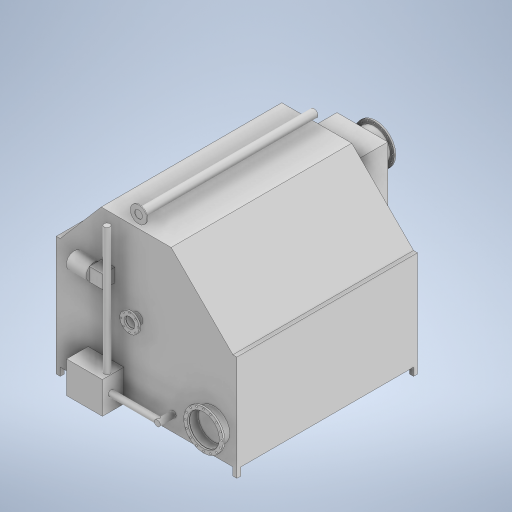
# Autodesk Inventor part: dummy
Saved by Autodesk Inventor 2023.1 (Build 271208000, 208)
## iProperties
Created: 2023-11-07
Part Number: dummy
Material: Generic
Document SubType Name: Modeling
Designer: admin
Density: 1 g/cm^3
Appearance: Default
Author: admin
Autodesk Inventor part; units mm, degrees
ref_plane "YZ Plane" through (0, 0, 0) normal (1, 0, 0) x (0, 1, 0)
ref_plane "XZ Plane" through (0, 0, 0) normal (0, 1, 0) x (-1, 0, 0)
ref_plane "XY Plane" through (0, 0, 0) normal (0, 0, 1) x (1, 0, 0)
sketch "Sketch1" plane through (0, 0, 0) normal (0, 0, 1) x (1, 0, 0)
  line L0 (-1135, 100) -> (1135, 100)
  line L1 (1135, 100) -> (1135, 1320)
  line L2 (1135, 1320) -> (-1135, 1320)
  line L3 (-1135, 1320) -> (-1135, 100)
  line L4 (-1135, 1320) -> (-1135, 1500)
  line L5 (-571.0934, 2100) -> (308.9066, 2100)
  line L6 (-1135, 1500) -> (-1085, 1500)
  line L7 (-1085, 1500) -> (-571.0934, 2100)
  line L8 (308.9066, 2100) -> (1085, 1320)
  point P0 (0, 0)
  point P1 (0, 100)
  dimension "d0" = 2270
  dimension "d1" = 100
  dimension "d2" = 1220
  dimension "d3" = 1400
  dimension "d4" = 880
  dimension "d5" = 50
  dimension "d6" = 50
  dimension "d7" = 2000
  dimension "d8" = 790
  dimension "d9" = 1100.3277
  constraints: 18 end point, 3 horizontal, 2 parallel, 1 midpoint, 1 perpendicular, 1 point on line, 1 vertical, 1 vertical alignment
  measures "d0" distance of L1.end L2.end
  measures "d1" distance from line of point (0, 0) L0
  measures "d2" distance of L0.end L1.end
  measures "d3" distance from line of L0 L4.end
  measures "d4" distance of L5.start L5.end
  measures "d5" distance of L4.end L6.end
  measures "d6" distance of L1.end L8.end
  measures "d7" distance between parallel lines of L0 L5
  measures "d8" distance of L6.end L5.start
  measures "d9" distance of L5.end L8.end
extrude "Extrusion1" add sketch "Sketch1" along normal mid plane 2270
sketch "Sketch2" plane through (-1135, 100, 1135) normal (0, -1, 0) x (1, 0, 0)
  line L0 (2270, -2270) -> (2270, 0) projected
  line L1 (0, 0) -> (2270, 0) projected
  line L2 (0, -2270) -> (0, 0) projected
  line L3 (2270, -2270) -> (0, -2270) projected
  line L4 (2270, 0) -> (2220, 0) projected
  line L5 (2270, 0) -> (2220, 0)
  line L6 (2220, 0) -> (2220, -50)
  line L7 (2220, -50) -> (2270, -50)
  line L8 (2270, -50) -> (2270, 0)
  line L9 (2220, -2270) -> (2270, -2270) projected
  line L10 (2270, -2270) -> (2220, -2270)
  line L11 (2220, -2270) -> (2220, -2220)
  line L12 (2220, -2220) -> (2270, -2220)
  line L13 (2270, -2220) -> (2270, -2270)
  line L14 (0, -2270) -> (50, -2270)
  line L15 (50, -2270) -> (50, -2220)
  line L16 (50, -2220) -> (0, -2220)
  line L17 (0, -2220) -> (0, -2270)
  line L18 (0, 0) -> (50, 0)
  line L19 (50, 0) -> (50, -50)
  line L20 (50, -50) -> (0, -50)
  line L21 (0, -50) -> (0, 0)
  line L22 (1160, -1110) -> (1110, -1110)
  line L23 (1110, -1110) -> (1110, -1160)
  line L24 (1110, -1160) -> (1160, -1160)
  line L25 (1160, -1160) -> (1160, -1110)
  line L26 (1160, -1110) -> (1110, -1160) construction
  line L27 (1110, -1110) -> (1160, -1160) construction
  point P0 (1135, -1135)
  point P1 (0, -2220)
  point P2 (50, -2270)
  dimension "d12" = 50
  dimension "d13" = 50
  constraints: 44 end point, 10 parallel, 8 equal length, 5 horizontal, 5 perpendicular, 2 midpoint, 1 point on line
  measures "d12" distance of L7.end L6.end
  measures "d13" distance of L5.end L6.end
extrude "Extrusion2" add sketch "Sketch2" along normal blind 100 contours L3 L11 L12 L0 | L7 L6 L1 L0 | L3 L2 L16 L15 | L19 L20 L2 L1 | L25 L24 L23 L22
sketch "Sketch3" plane through (0, 0, 1135) normal (0, 0, 1) x (1, 0, 0)
  circle A0 centre (845, 445) radius 200
  line L0 (-1085, 100) -> (1085, 100) projected
  circle A1 centre (845, 445) radius 195
  line L1 (1135, 1320) -> (1135, 0) projected
  line L2 (650, 640) -> (1040, 640) construction
  line L3 (1040, 640) -> (1040, 250) construction
  line L4 (1040, 250) -> (650, 250) construction
  line L5 (650, 250) -> (650, 640) construction
  point P0 (0, 0)
  point P1 (1135, 660)
  dimension "d18" = 400
  dimension "d19" = 390
  dimension "d20" = 95
  dimension "d21" = 485
  dimension "d22" = 150
  dimension "d23" = 540
  constraints: 8 end point, 4 tangent, 2 centre point, 2 parallel, 1 horizontal, 1 midpoint, 1 perpendicular
  measures "d18" diameter of A0
  measures "d19" diameter of A1
  measures "d20" distance between parallel lines of L1 L3
  measures "d21" distance from line of L5 point (1135, 660)
  measures "d22" distance between parallel lines of L0 L4
  measures "d23" distance between parallel lines of L0 L2
extrude "Extrusion3" add sketch "Sketch3" along normal blind 110
sketch "Sketch4" plane through (0, 0, 1135) normal (0, 0, 1) x (1, 0, 0)
  line L0 (1135, 1320) -> (1085, 1320) projected
  line L1 (1085, 1320) -> (308.9066, 2100) projected
  line L2 (308.9066, 2100) -> (-571.0934, 2100) projected
  line L3 (-571.0934, 2100) -> (-1085, 1500) projected
  line L4 (-1085, 1500) -> (-1135, 1500) projected
  line L5 (-1135, 1500) -> (-1135, 0) projected
  line L6 (-1085, 0) -> (-1135, 0) projected
  line L7 (-1085, 100) -> (-1085, 0) projected
  line L8 (-1085, 100) -> (1085, 100) projected
  line L9 (1085, 100) -> (1085, 0) projected
  line L10 (1135, 0) -> (1085, 0) projected
  line L11 (1135, 1320) -> (1135, 0) projected
  circle A0 centre (845, 445) radius 200 projected
  circle A1 centre (-115, 1120) radius 62.5
  line L12 (-177.5, 1182.5) -> (-52.5, 1182.5) construction
  line L13 (-52.5, 1182.5) -> (-52.5, 1057.5) construction
  line L14 (-52.5, 1057.5) -> (-177.5, 1057.5) construction
  line L15 (-177.5, 1057.5) -> (-177.5, 1182.5) construction
  circle A2 centre (-115, 1120) radius 67.5
  line L16 (25, 0) -> (-25, 0) projected
  point P0 (0, 0)
  point P1 (0, 0)
  dimension "d26" = 125
  dimension "d28" = 957.5
  dimension "d30" = 1312.5
  dimension "d31" = 5
  dimension "d134" = 1020
  dimension "d135" = 1120
  constraints: 8 end point, 4 tangent, 2 centre point, 2 parallel, 1 horizontal, 1 midpoint, 1 perpendicular
  measures "d26" diameter of A1
  measures "d28" distance between parallel lines of L8 L14
  measures "d30" distance between parallel lines of L11 L15
  measures "d31" radial gap between concentric circles of A1 A2
  measures "d134" distance from line of A1.centre L5
  measures "d135" vertical distance of A1.centre point (0, 0)
extrude "Extrusion4" add sketch "Sketch4" along normal blind 80 contours A2
sketch "Sketch5" plane through (845, 445, 1245) normal (0, 0, 1) x (1, 0, 0)
  circle A0 centre (0, 0) radius 200 projected
  circle A1 centre (0, 0) radius 250
  circle A2 centre (0, 0) radius 230 construction
  circle A3 centre (0, 230) radius 11
  circle A4 centre (-88.0172, 212.4923) radius 11
  circle A5 centre (-162.6346, 162.6346) radius 11
  circle A6 centre (-212.4923, 88.0172) radius 11
  circle A7 centre (-230, 0) radius 11
  circle A8 centre (-212.4923, -88.0172) radius 11
  circle A9 centre (-162.6346, -162.6346) radius 11
  circle A10 centre (-88.0172, -212.4923) radius 11
  circle A11 centre (0, -230) radius 11
  circle A12 centre (88.0172, -212.4923) radius 11
  circle A13 centre (162.6346, -162.6346) radius 11
  circle A14 centre (212.4923, -88.0172) radius 11
  circle A15 centre (230, 0) radius 11
  circle A16 centre (212.4923, 88.0172) radius 11
  circle A17 centre (162.6346, 162.6346) radius 11
  circle A18 centre (88.0172, 212.4923) radius 11
  point P0 (-845, -445)
  dimension "d35" = 460
  dimension "d34" = 500
  dimension "d36" = 22
  dimension "d39" = 360
  constraints: 17 centre point, 2 vertical alignment, 1 coincident, 35 other
  measures "d34" diameter of A1
  measures "d36" diameter of A3
extrude "Extrusion5" add sketch "Sketch5" along normal blind 20
sketch "Sketch6" plane through (-115, 1120, 1215) normal (0, 0, 1) x (1, 0, 0)
  circle A0 centre (0, 0) radius 67.5 projected
  circle A1 centre (0, 0) radius 122.5
  circle A2 centre (0, 0) radius 105 construction
  circle A3 centre (0, 105) radius 9
  circle A4 centre (-74.2462, 74.2462) radius 9
  circle A5 centre (-105, 0) radius 9
  circle A6 centre (-74.2462, -74.2462) radius 9
  circle A7 centre (0, -105) radius 9
  circle A8 centre (74.2462, -74.2462) radius 9
  circle A9 centre (105, 0) radius 9
  circle A10 centre (74.2462, 74.2462) radius 9
  point P0 (115, -1120)
  dimension "d44" = 210
  dimension "d43" = 245
  dimension "d45" = 18
  dimension "d48" = 360
  constraints: 9 centre point, 2 coincident, 2 vertical alignment, 19 other
  measures "d43" diameter of A1
  measures "d45" diameter of A3
extrude "Extrusion6" add sketch "Sketch6" along normal blind 20
sketch "Sketch7" plane through (0, 0, 1135) normal (0, 0, 1) x (1, 0, 0)
  circle A0 centre (845, 445) radius 200 projected
  line L0 (1135, 1320) -> (1085, 1320) projected
  line L1 (1085, 1320) -> (308.9066, 2100) projected
  line L2 (308.9066, 2100) -> (-571.0934, 2100) projected
  line L3 (-571.0934, 2100) -> (-1085, 1500) projected
  line L4 (-1085, 1500) -> (-1135, 1500) projected
  line L5 (-1135, 1500) -> (-1135, 0) projected
  line L6 (-1085, 0) -> (-1135, 0) projected
  line L7 (-1085, 100) -> (-1085, 0) projected
  line L8 (-1085, 100) -> (1085, 100) projected
  line L9 (1085, 100) -> (1085, 0) projected
  line L10 (1135, 0) -> (1085, 0) projected
  line L11 (1135, 1320) -> (1135, 0) projected
  circle A1 centre (-115, 1120) radius 67.5 projected
  line L12 (-570, 1530) -> (-400, 1530)
  line L13 (-400, 1530) -> (-400, 1360)
  line L14 (-400, 1360) -> (-570, 1360)
  line L15 (-570, 1360) -> (-570, 1530)
  line L16 (-570, 1530) -> (-400, 1360) construction
  line L17 (-400, 1530) -> (-570, 1360) construction
  point P0 (0, 0)
  point P1 (-485, 1445)
  dimension "d52" = 170
  dimension "d53" = 170
  dimension "d54" = 1535
  dimension "d55" = 1260
  constraints: 12 end point, 2 midpoint, 2 parallel, 1 horizontal, 1 perpendicular
  measures "d52" distance of L13.end L14.end
  measures "d53" distance of L12.end L13.end
  measures "d54" distance between parallel lines of L13 L11
  measures "d55" distance between parallel lines of L14 L8
extrude "Extrusion7" add sketch "Sketch7" along normal blind 150 contours L12 L13 L14 L15
sketch "Sketch8" plane through (-570, 1360, 1135) normal (-1, 0, 0) x (0, 0, 1)
  line L0 (0, 0) -> (0, 170) projected
  line L1 (0, 0) -> (150, 0) projected
  line L2 (150, 170) -> (150, 0) projected
  line L3 (0, 170) -> (150, 170) projected
  circle A0 centre (90, 85) radius 100
  point P0 (-1135, -1360)
  dimension "d58" = 200
  dimension "d59" = 90
  constraints: 1 centre point
  measures "d58" diameter of A0
  measures "d59" distance from line of A0.centre L0
extrude "Extrusion8" add sketch "Sketch8" along normal blind 250 contours A0 L0 | L0 A0 L3 L2 L1 | L1 A0 | A0 L3 | L2 A0
sketch "Sketch9" plane through (0, 0, 1135) normal (0, 0, 1) x (1, 0, 0)
  line L0 (-820, 1488.589) -> (-570, 1488.589) projected
  line L1 (-570, 1488.589) -> (-570, 1530) projected
  line L2 (-570, 1530) -> (-400, 1530) projected
  line L3 (-400, 1530) -> (-400, 1360) projected
  line L4 (-400, 1360) -> (-570, 1360) projected
  line L5 (-570, 1360) -> (-570, 1401.411) projected
  line L6 (-570, 1401.411) -> (-820, 1401.411) projected
  line L7 (-820, 1401.411) -> (-820, 1488.589) projected
  circle A0 centre (845, 445) radius 200 projected
  line L8 (1135, 1320) -> (1085, 1320) projected
  line L9 (1085, 1320) -> (308.9066, 2100) projected
  line L10 (308.9066, 2100) -> (-571.0934, 2100) projected
  line L11 (-571.0934, 2100) -> (-1085, 1500) projected
  line L12 (-1085, 1500) -> (-1135, 1500) projected
  line L13 (-1135, 1500) -> (-1135, 0) projected
  line L14 (-1085, 0) -> (-1135, 0) projected
  line L15 (-1085, 100) -> (-1085, 0) projected
  line L16 (-1085, 100) -> (1085, 100) projected
  line L17 (1085, 100) -> (1085, 0) projected
  line L18 (1135, 0) -> (1085, 0) projected
  line L19 (1135, 1320) -> (1135, 0) projected
  circle A1 centre (-115, 1120) radius 67.5 projected
  line L20 (-735, 500) -> (-285, 500)
  line L21 (-285, 500) -> (-285, 100)
  line L22 (-285, 100) -> (-735, 100)
  line L23 (-735, 100) -> (-735, 500)
  line L24 (-735, 500) -> (-285, 100) construction
  line L25 (-285, 500) -> (-735, 100) construction
  line L26 (-1085, 100) -> (1085, 100) projected
  point P0 (0, 0)
  point P1 (-25, 0)
  point P2 (-510, 300)
  dimension "d62" = 400
  dimension "d63" = 400
  dimension "d64" = 450
  constraints: 12 end point, 2 midpoint, 2 parallel, 1 collinear, 1 horizontal, 1 perpendicular
  measures "d62" distance of L20.end L21.end
  measures "d63" distance between parallel lines of L23 L13
  measures "d64" distance of L20.start L20.end
extrude "Extrusion9" add sketch "Sketch9" along normal blind 270 contours L16 L23 L20 L21
sketch "Sketch10" plane through (0, 0, 1135) normal (0, 0, 1) x (1, 0, 0)
  line L0 (-285, 500) -> (-285, 100) projected
  line L1 (-285, 100) -> (1085, 100) projected
  line L2 (1085, 100) -> (1085, 0) projected
  line L3 (1135, 0) -> (1085, 0) projected
  line L4 (1135, 1320) -> (1135, 0) projected
  line L5 (1135, 1320) -> (1085, 1320) projected
  line L6 (1085, 1320) -> (308.9066, 2100) projected
  line L7 (308.9066, 2100) -> (-571.0934, 2100) projected
  line L8 (-571.0934, 2100) -> (-1085, 1500) projected
  line L9 (-1085, 1500) -> (-1135, 1500) projected
  line L10 (-1135, 1500) -> (-1135, 0) projected
  line L11 (-1085, 0) -> (-1135, 0) projected
  line L12 (-1085, 100) -> (-1085, 0) projected
  line L13 (-1085, 100) -> (-735, 100) projected
  line L14 (-735, 100) -> (-735, 500) projected
  line L15 (-735, 500) -> (-285, 500) projected
  line L16 (-820, 1488.589) -> (-570, 1488.589) projected
  line L17 (-570, 1488.589) -> (-570, 1530) projected
  line L18 (-570, 1530) -> (-400, 1530) projected
  line L19 (-400, 1530) -> (-400, 1360) projected
  line L20 (-400, 1360) -> (-570, 1360) projected
  line L21 (-570, 1360) -> (-570, 1401.411) projected
  line L22 (-570, 1401.411) -> (-820, 1401.411) projected
  line L23 (-820, 1401.411) -> (-820, 1488.589) projected
  circle A0 centre (845, 445) radius 200 projected
  circle A1 centre (-115, 1120) radius 67.5 projected
  circle A2 centre (335, 300) radius 37.5
  point P0 (0, 0)
  dimension "d67" = 75
  dimension "d68" = 200
  dimension "d69" = 800
  constraints: 1 centre point
  measures "d67" diameter of A2
  measures "d68" distance from line of L1 A2.centre
  measures "d69" distance from line of A2.centre L4
extrude "Extrusion10" add sketch "Sketch10" along normal blind 200 contours A2
sketch "Sketch11" plane through (0, 0, 0) normal (0, 0, 1) x (1, 0, 0)
  circle A0 centre (-131.0934, 2225) radius 50
  line L0 (-371.0458, 2175) -> (-85.5673, 2175) construction
  line L1 (308.9066, 2100) -> (-571.0934, 2100) projected
  point P0 (0, 0)
  point P1 (-131.0934, 2100)
  dimension "d72" = 100
  dimension "d73" = 75
  constraints: 2 end point, 1 centre point, 1 horizontal, 1 midpoint, 1 tangent, 1 vertical alignment
  measures "d72" diameter of A0
  measures "d73" distance between parallel lines of L1 L0
extrude "Extrusion11" add sketch "Sketch11" along normal mid plane 2200
sketch "Sketch12" plane through (-131.0934, 2225, 1100) normal (0, 0, 1) x (1, 0, 0)
  circle A0 centre (0, 0) radius 50 projected
  circle A1 centre (0, 0) radius 105
  point P0 (131.0934, -2225)
  dimension "d76" = 210
  constraints: 1 centre point, 1 coincident
  measures "d76" diameter of A1
extrude "Extrusion12" add sketch "Sketch12" along normal mid plane 10
sketch "Sketch13" plane through (0, 0, -1135) normal (0, 0, -1) x (-1, 0, 0)
  line L0 (-1085, 1320) -> (-1135, 1320) projected
  line L1 (-1135, 1320) -> (-1135, 0) projected
  line L2 (-1085, 0) -> (-1135, 0) projected
  line L3 (-1085, 100) -> (-1085, 0) projected
  line L4 (-1085, 100) -> (1085, 100) projected
  line L5 (1085, 100) -> (1085, 0) projected
  line L6 (1135, 0) -> (1085, 0) projected
  line L7 (1135, 1500) -> (1135, 0) projected
  line L8 (1135, 1500) -> (1085, 1500) projected
  line L9 (1085, 1500) -> (571.0934, 2100) projected
  line L10 (571.0934, 2100) -> (-308.9066, 2100) projected
  line L11 (-308.9066, 2100) -> (-1085, 1320) projected
  line L12 (-300, 860) -> (575, 860)
  line L13 (575, 860) -> (575, 810)
  line L14 (575, 810) -> (-300, 810)
  line L15 (-300, 810) -> (-300, 860)
  line L16 (-300, 860) -> (575, 810) construction
  line L17 (575, 860) -> (-300, 810) construction
  point P0 (0, 0)
  point P1 (137.5, 835)
  dimension "d79" = 875
  dimension "d80" = 50
  dimension "d81" = 760
  dimension "d82" = 560
  constraints: 12 end point, 2 midpoint, 2 parallel, 1 horizontal, 1 perpendicular
  measures "d79" distance of L13.end L14.end
  measures "d80" distance of L12.end L13.end
  measures "d81" distance between parallel lines of L12 L4
  measures "d82" distance between parallel lines of L13 L7
extrude "Extrusion13" add sketch "Sketch13" along normal blind 580 contours L12 L13 L14 L15
sketch "Sketch14" plane through (-575, 860, -1135) normal (0, 1, 0) x (1, 0, 0)
  line L0 (875, 0) -> (0, 0) projected
  line L1 (875, 0) -> (875, 580) projected
  line L2 (0, 580) -> (875, 580) projected
  line L3 (0, 0) -> (0, 580) projected
  line L4 (757.5, 130) -> (117.5, 130)
  line L5 (117.5, 130) -> (117.5, 580)
  line L6 (117.5, 580) -> (757.5, 580)
  line L7 (757.5, 580) -> (757.5, 130)
  line L8 (757.5, 130) -> (117.5, 580) construction
  line L9 (117.5, 130) -> (757.5, 580) construction
  line L10 (0, 580) -> (875, 580) projected
  point P0 (575, -1135)
  point P1 (437.5, 355)
  point P2 (437.5, 580)
  point P3 (437.5, 580)
  point P4 (757.5, 580)
  point P5 (117.5, 580)
  dimension "d85" = 640
  dimension "d86" = 450
  constraints: 12 end point, 4 midpoint, 2 parallel, 1 coincident, 1 collinear, 1 horizontal, 1 perpendicular
  measures "d85" distance of L5.end L6.end
  measures "d86" distance of L4.end L5.end
extrude "Extrusion14" add sketch "Sketch14" along normal blind 900 contours L7 L4 L5 L2
sketch "Sketch15" plane through (0, 0, -1715) normal (0, 0, -1) x (-1, 0, 0)
  line L0 (-300, 810) -> (575, 810) projected
  line L1 (575, 810) -> (575, 860) projected
  line L2 (575, 860) -> (457.5, 860) projected
  line L3 (457.5, 860) -> (457.5, 1760) construction
  line L4 (-182.5, 1760) -> (457.5, 1760) construction
  line L5 (-182.5, 860) -> (-182.5, 1760) construction
  line L6 (-182.5, 860) -> (-300, 860) projected
  line L7 (-300, 860) -> (-300, 810) projected
  circle A0 centre (137.5, 1500) radius 200
  line L8 (-182.5, 1700) -> (457.5, 1700) construction
  line L9 (457.5, 860) -> (457.5, 1760) projected
  circle A1 centre (137.5, 1500) radius 250 construction
  point P0 (0, 0)
  point P1 (137.5, 1760)
  dimension "d89" = 400
  dimension "d90" = 60
  dimension "d91" = 500
  constraints: 2 centre point, 2 end point, 2 point on line, 1 coincident, 1 midpoint, 1 perpendicular, 1 tangent, 1 vertical alignment
  measures "d89" diameter of A0
  measures "d90" distance between parallel lines of L4 L8
  measures "d91" diameter of A1
extrude "Extrusion15" add sketch "Sketch15" along normal blind 150
sketch "Sketch16" plane through (-137.5, 1500, -1865) normal (0, 0, -1) x (-1, 0, 0)
  circle A0 centre (0, 0) radius 200 construction
  circle A1 centre (0, 0) radius 250
  circle A2 centre (0, 0) radius 175
  circle A3 centre (0, 0) radius 230 construction
  circle A4 centre (0, 230) radius 11
  circle A5 centre (-88.0172, 212.4923) radius 11
  circle A6 centre (-162.6346, 162.6346) radius 11
  circle A7 centre (-212.4923, 88.0172) radius 11
  circle A8 centre (-230, 0) radius 11
  circle A9 centre (-212.4923, -88.0172) radius 11
  circle A10 centre (-162.6346, -162.6346) radius 11
  circle A11 centre (-88.0172, -212.4923) radius 11
  circle A12 centre (0, -230) radius 11
  circle A13 centre (88.0172, -212.4923) radius 11
  circle A14 centre (162.6346, -162.6346) radius 11
  circle A15 centre (212.4923, -88.0172) radius 11
  circle A16 centre (230, 0) radius 11
  circle A17 centre (212.4923, 88.0172) radius 11
  circle A18 centre (162.6346, 162.6346) radius 11
  circle A19 centre (88.0172, 212.4923) radius 11
  point P0 (-137.5, -1500)
  dimension "d96" = 460
  dimension "d94" = 500
  dimension "d95" = 350
  dimension "d97" = 22
  dimension "d100" = 360
  constraints: 18 centre point, 3 coincident, 2 vertical alignment, 35 other
  measures "d94" diameter of A1
  measures "d95" diameter of A2
  measures "d97" diameter of A4
extrude "Extrusion16" add sketch "Sketch16" along normal blind 20
sketch "Sketch17" plane through (-457.5, 860, -1265) normal (0, 0, 1) x (1, 0, 0)
  circle A0 centre (320, 640) radius 200 construction
  line L0 (757.5, -50) -> (-117.5, -50) projected
  line L1 (-117.5, -50) -> (-117.5, 0) projected
  line L2 (-117.5, 0) -> (0, 0) projected
  line L3 (0, 0) -> (0, 900) projected
  line L4 (640, 900) -> (0, 900) projected
  line L5 (640, 0) -> (640, 900) projected
  line L6 (640, 0) -> (757.5, 0) projected
  line L7 (757.5, 0) -> (757.5, -50) projected
  circle A1 centre (320, 300) radius 200
  point P0 (457.5, -860)
  dimension "d104" = 400
  dimension "d105" = 300
  constraints: 1 centre point, 1 vertical alignment
  measures "d104" diameter of A1
  measures "d105" distance from line of L6 A1.centre
extrude "Extrusion17" add sketch "Sketch17" along normal up to surface (130 mm away) contours A1
sketch "Sketch18" plane through (0, 0, -1135) normal (0, 0, -1) x (-1, 0, 0)
  circle A0 centre (-335, 310) radius 55
  line L0 (-1135, 1320) -> (-1135, 0) projected
  line L1 (-1085, 100) -> (1085, 100) projected
  point P0 (0, 0)
  dimension "d108" = 110
  dimension "d109" = 800
  dimension "d110" = 210
  constraints: 1 centre point
  measures "d108" diameter of A0
  measures "d109" distance from line of L0 A0.centre
  measures "d110" distance from line of A0.centre L1
extrude "Extrusion18" add sketch "Sketch18" along normal blind 60
sketch "Sketch19" plane through (335, 310, -1195) normal (0, 0, -1) x (-1, 0, 0)
  circle A0 centre (0, 0) radius 55 projected
  circle A1 centre (0, 0) radius 110
  circle A2 centre (0, 90) radius 9
  circle A3 centre (0, 0) radius 90 construction
  circle A4 centre (-63.6396, 63.6396) radius 9
  circle A5 centre (-90, 0) radius 9
  circle A6 centre (-63.6396, -63.6396) radius 9
  circle A7 centre (0, -90) radius 9
  circle A8 centre (63.6396, -63.6396) radius 9
  circle A9 centre (90, 0) radius 9
  circle A10 centre (63.6396, 63.6396) radius 9
  point P0 (335, -310)
  dimension "d115" = 180
  dimension "d113" = 220
  dimension "d114" = 18
  dimension "d120" = 360
  constraints: 9 centre point, 2 coincident, 2 vertical alignment, 19 other
  measures "d113" diameter of A1
  measures "d114" diameter of A2
extrude "Extrusion19" add sketch "Sketch19" along normal blind 10
sketch "Sketch20" plane through (-457.5, 860, -1715) normal (-1, 0, 0) x (0, 0, 1)
  line L0 (450, 0) -> (0, 0) projected
  line L1 (450, 0) -> (450, 900) projected
  line L2 (0, 900) -> (450, 900) projected
  line L3 (0, 0) -> (0, 900) projected
  circle A0 centre (225, 760) radius 80
  point P0 (1715, -860)
  point P1 (225, 900)
  dimension "d122" = 160
  dimension "d123" = 140
  constraints: 1 centre point, 1 midpoint, 1 vertical alignment
  measures "d122" diameter of A0
  measures "d123" distance from line of L2 A0.centre
extrude "Extrusion20" add sketch "Sketch20" along normal blind 330 contours A0
sketch "Sketch21" plane through (0, 0, -1135) normal (0, 0, -1) x (-1, 0, 0)
  line L0 (787.5, 1540) -> (787.5, 1700) projected
  line L1 (457.5, 1700) -> (457.5, 1540) projected
  circle A0 centre (717.5, 1620) radius 70
  point P0 (0, 0)
  point P1 (457.5, 1620)
  dimension "d126" = 140
  constraints: 1 centre point, 1 horizontal alignment, 1 midpoint, 1 tangent
  measures "d126" diameter of A0
extrude "Extrusion21" add sketch "Sketch21" along normal blind 330
sketch "Sketch22" plane through (-285, 100, 1135) normal (1, 0, 0) x (0, 0, -1)
  line L0 (-200, 237.5) -> (-200, 162.5) projected
  line L1 (0, 162.5) -> (0, 237.5) projected
  line L2 (0, 237.5) -> (-200, 237.5) projected
  line L3 (0, 162.5) -> (-200, 162.5) projected
  circle A0 centre (-162.5, 200) radius 37.5
  point P0 (1135, -100)
  constraints: 3 tangent, 1 centre point
extrude "Extrusion22" add sketch "Sketch22" along normal up to surface contours A0
sketch "Sketch23" plane through (-735, 500, 1135) normal (0, 1, 0) x (1, 0, 0)
  circle A0 centre (400, -162.5) radius 37.5
  line L0 (0, 0) -> (450, 0) projected
  line L1 (0, 0) -> (0, -270) projected
  line L2 (450, -270) -> (0, -270) projected
  line L3 (450, 0) -> (450, -270) projected
  line L4 (450, -200) -> (1032.5, -200) projected
  line L5 (450, -125) -> (1032.5, -125) projected
  point P0 (735, 1135)
  point P1 (450, -135)
  dimension "d131" = 50
  constraints: 2 tangent, 1 centre point, 1 midpoint
  measures "d131" horizontal distance of point (450, -135) A0.centre
extrude "Extrusion23" add sketch "Sketch23" along normal up to surface (1600 mm away) contours A0
body "Solid1"
